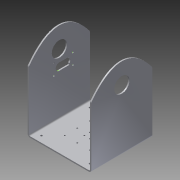
# Autodesk Inventor part: U Arms
Saved by Autodesk Inventor 2015 (Build 190159000, 159)
## iProperties
Created: 2014-05-20
Part Number: U Arms
Material: Aluminum 6061
Document SubType Name: Sheet Metal
Designer: seaha_000
Density: 2.71 g/cm^3
Sheet Metal Rule: 1/8in Aluminium
Sheet Metal Width: 6.000 in
Sheet Metal Length: 21.815 in
Sheet Metal Area: 130.893 in^2
Appearance: Aluminum - Flat
Flat Pattern Width: 15.24 cm
Flat Pattern Length: 55.4113 cm
Flat Pattern Area: 844.469 cm^2
Mass: 656.228 g
Surface Area: 1584.51 cm^2
Volume: 242.15 cm^3
Author: seaha_000
Autodesk Inventor part; units mm, degrees
ref_plane "YZ Plane" through (0, 0, 0) normal (1, 0, 0) x (0, 1, 0)
ref_plane "XZ Plane" through (0, 0, 0) normal (0, 1, 0) x (-1, 0, 0)
ref_plane "XY Plane" through (0, 0, 0) normal (0, 0, 1) x (1, 0, 0)
sketch "Sketch3" plane through (0, 0, 0) normal (0, 1, 0) x (-1, 0, 0)
  line L0 (-79.375, 76.2) -> (79.375, 76.2)
  line L1 (79.375, 76.2) -> (79.375, -76.2)
  line L2 (79.375, -76.2) -> (-79.375, -76.2)
  line L3 (-79.375, -76.2) -> (-79.375, 76.2)
  line L4 (-79.375, 76.2) -> (79.375, -76.2) construction
  line L5 (79.375, 76.2) -> (-79.375, -76.2) construction
  arc A0 (-19.05, -1.8288) -> (-19.05, 1.8288) centre (-19.05, 0) ccw
  arc A1 (-19.05, 1.8288) -> (-19.05, -1.8288) centre (-19.05, 0) ccw
  arc A2 (-6.9148, -8.7436) -> (-6.9148, -5.086) centre (-6.9148, -6.9148) ccw
  arc A3 (-6.9148, -5.086) -> (-6.9148, -8.7436) centre (-6.9148, -6.9148) ccw
  arc A4 (-6.9148, 5.086) -> (-6.9148, 8.7436) centre (-6.9148, 6.9148) ccw
  arc A5 (-6.9148, 8.7436) -> (-6.9148, 5.086) centre (-6.9148, 6.9148) ccw
  arc A6 (6.9148, 5.086) -> (6.9148, 8.7436) centre (6.9148, 6.9148) ccw
  arc A7 (6.9148, 8.7436) -> (6.9148, 5.086) centre (6.9148, 6.9148) ccw
  arc A8 (0, 17.2212) -> (0, 20.8788) centre (0, 19.05) ccw
  arc A9 (0, 20.8788) -> (0, 17.2212) centre (0, 19.05) ccw
  arc A10 (19.05, -1.8288) -> (19.05, 1.8288) centre (19.05, 0) ccw
  arc A11 (19.05, 1.8288) -> (19.05, -1.8288) centre (19.05, 0) ccw
  arc A12 (6.9148, -8.7436) -> (6.9148, -5.086) centre (6.9148, -6.9148) ccw
  arc A13 (6.9148, -5.086) -> (6.9148, -8.7436) centre (6.9148, -6.9148) ccw
  arc A14 (0, -20.8788) -> (0, -17.2212) centre (0, -19.05) ccw
  arc A15 (0, -17.2212) -> (0, -20.8788) centre (0, -19.05) ccw
  arc A16 (0, -46.236) -> (0, -42.664) centre (0, -44.45) ccw
  arc A17 (0, -42.664) -> (0, -46.236) centre (0, -44.45) ccw
  arc A18 (0, -33.536) -> (0, -29.964) centre (0, -31.75) ccw
  arc A19 (0, -29.964) -> (0, -33.536) centre (0, -31.75) ccw
  arc A20 (0, -11.565) -> (0, -7.993) centre (0, -9.779) ccw
  arc A21 (0, -7.993) -> (0, -11.565) centre (0, -9.779) ccw
  arc A22 (13.4704, -15.2564) -> (13.4704, -11.6844) centre (13.4704, -13.4704) ccw
  arc A23 (13.4704, -11.6844) -> (13.4704, -15.2564) centre (13.4704, -13.4704) ccw
  arc A24 (22.4506, -24.2366) -> (22.4506, -20.6646) centre (22.4506, -22.4506) ccw
  arc A25 (22.4506, -20.6646) -> (22.4506, -24.2366) centre (22.4506, -22.4506) ccw
  arc A26 (31.4309, -33.2169) -> (31.4309, -29.6449) centre (31.4309, -31.4309) ccw
  arc A27 (31.4309, -29.6449) -> (31.4309, -33.2169) centre (31.4309, -31.4309) ccw
  arc A28 (44.45, -1.786) -> (44.45, 1.786) centre (44.45, 0) ccw
  arc A29 (44.45, 1.786) -> (44.45, -1.786) centre (44.45, 0) ccw
  arc A30 (31.75, -1.786) -> (31.75, 1.786) centre (31.75, 0) ccw
  arc A31 (31.75, 1.786) -> (31.75, -1.786) centre (31.75, 0) ccw
  arc A32 (9.779, -1.786) -> (9.779, 1.786) centre (9.779, 0) ccw
  arc A33 (9.779, 1.786) -> (9.779, -1.786) centre (9.779, 0) ccw
  arc A34 (13.4704, 11.6844) -> (13.4704, 15.2564) centre (13.4704, 13.4704) ccw
  arc A35 (13.4704, 15.2564) -> (13.4704, 11.6844) centre (13.4704, 13.4704) ccw
  arc A36 (22.4506, 20.6646) -> (22.4506, 24.2366) centre (22.4506, 22.4506) ccw
  arc A37 (22.4506, 24.2366) -> (22.4506, 20.6646) centre (22.4506, 22.4506) ccw
  arc A38 (31.4309, 29.6449) -> (31.4309, 33.2169) centre (31.4309, 31.4309) ccw
  arc A39 (31.4309, 33.2169) -> (31.4309, 29.6449) centre (31.4309, 31.4309) ccw
  arc A40 (0, 42.664) -> (0, 46.236) centre (0, 44.45) ccw
  arc A41 (0, 46.236) -> (0, 42.664) centre (0, 44.45) ccw
  arc A42 (0, 29.964) -> (0, 33.536) centre (0, 31.75) ccw
  arc A43 (0, 33.536) -> (0, 29.964) centre (0, 31.75) ccw
  arc A44 (0, 7.993) -> (0, 11.565) centre (0, 9.779) ccw
  arc A45 (0, 11.565) -> (0, 7.993) centre (0, 9.779) ccw
  arc A46 (-13.4704, 11.6844) -> (-13.4704, 15.2564) centre (-13.4704, 13.4704) ccw
  arc A47 (-13.4704, 15.2564) -> (-13.4704, 11.6844) centre (-13.4704, 13.4704) ccw
  arc A48 (-22.4506, 20.6646) -> (-22.4506, 24.2366) centre (-22.4506, 22.4506) ccw
  arc A49 (-22.4506, 24.2366) -> (-22.4506, 20.6646) centre (-22.4506, 22.4506) ccw
  arc A50 (-31.4309, 29.6449) -> (-31.4309, 33.2169) centre (-31.4309, 31.4309) ccw
  arc A51 (-31.4309, 33.2169) -> (-31.4309, 29.6449) centre (-31.4309, 31.4309) ccw
  arc A52 (-44.45, -1.786) -> (-44.45, 1.786) centre (-44.45, 0) ccw
  arc A53 (-44.45, 1.786) -> (-44.45, -1.786) centre (-44.45, 0) ccw
  arc A54 (-31.75, -1.786) -> (-31.75, 1.786) centre (-31.75, 0) ccw
  arc A55 (-31.75, 1.786) -> (-31.75, -1.786) centre (-31.75, 0) ccw
  arc A56 (-9.779, -1.786) -> (-9.779, 1.786) centre (-9.779, 0) ccw
  arc A57 (-9.779, 1.786) -> (-9.779, -1.786) centre (-9.779, 0) ccw
  arc A58 (-13.4704, -15.2564) -> (-13.4704, -11.6844) centre (-13.4704, -13.4704) ccw
  arc A59 (-13.4704, -11.6844) -> (-13.4704, -15.2564) centre (-13.4704, -13.4704) ccw
  arc A60 (-22.4506, -24.2366) -> (-22.4506, -20.6646) centre (-22.4506, -22.4506) ccw
  arc A61 (-22.4506, -20.6646) -> (-22.4506, -24.2366) centre (-22.4506, -22.4506) ccw
  arc A62 (-31.4309, -33.2169) -> (-31.4309, -29.6449) centre (-31.4309, -31.4309) ccw
  arc A63 (-31.4309, -29.6449) -> (-31.4309, -33.2169) centre (-31.4309, -31.4309) ccw
  arc A64 (0, 50.038) -> (0, -50.038) centre (0, 0) ccw
  arc A65 (0, -50.038) -> (0, 50.038) centre (0, 0) ccw
  arc A66 (0, 6.35) -> (0, -6.35) centre (0, 0) ccw
  arc A67 (0, -6.35) -> (0, 6.35) centre (0, 0) ccw
  dimension "d185" = 158.75
  dimension "d186" = 152.4
  dimension "d187" = 1.786
  dimension "d188" = 1.786
  dimension "d189" = 1.786
  dimension "d190" = 1.786
  dimension "d191" = 1.786
  dimension "d192" = 1.786
  dimension "d193" = 1.786
  dimension "d194" = 1.8288
  dimension "d195" = 1.8288
  dimension "d196" = 1.786
  dimension "d197" = 1.786
  dimension "d198" = 1.786
  dimension "d199" = 1.8288
  dimension "d200" = 1.8288
  dimension "d201" = 1.786
  dimension "d202" = 1.786
  dimension "d203" = 1.8288
  dimension "d204" = 1.786
  dimension "d205" = 50.038
  dimension "d206" = 50.038
  dimension "d207" = 6.35
  dimension "d208" = 6.35
  dimension "d209" = 1.786
  dimension "d210" = 1.8288
  dimension "d211" = 1.786
  dimension "d212" = 1.786
  dimension "d213" = 1.8288
  dimension "d214" = 1.8288
  dimension "d215" = 1.786
  dimension "d216" = 1.786
  dimension "d217" = 1.786
  dimension "d218" = 1.8288
  dimension "d219" = 1.786
  dimension "d220" = 1.786
  dimension "d221" = 1.786
  dimension "d222" = 1.786
  dimension "d223" = 1.786
  dimension "d224" = 1.786
  dimension "d225" = 74.414
  dimension "d226" = 34.925
  dimension "d227" = 76.2
  dimension "d228" = 76.2
  dimension "d229" = 74.414
  dimension "d230" = 47.625
  dimension "d231" = 76.2
  dimension "d232" = 76.2
  dimension "d233" = 42.9831
  dimension "d234" = 47.9441
  dimension "d235" = 44.7691
  dimension "d236" = 44.7691
  dimension "d237" = 105.8449
  dimension "d238" = 47.9441
  dimension "d239" = 107.6309
  dimension "d240" = 107.6309
  dimension "d241" = 51.9634
  dimension "d242" = 56.9244
  dimension "d243" = 53.7494
  dimension "d244" = 53.7494
  dimension "d245" = 96.8646
  dimension "d246" = 56.9244
  dimension "d247" = 98.6506
  dimension "d248" = 98.6506
  measures "d185" distance of L1.end L2.end
  measures "d186" distance of L0.end L1.end
  measures "d187" radius of A29
  measures "d188" radius of A28
  measures "d189" radius of A30
  measures "d190" radius of A38
  measures "d191" radius of A26
  measures "d192" radius of A36
  measures "d193" radius of A24
  measures "d194" radius of A11
  measures "d195" radius of A10
  measures "d196" radius of A34
  measures "d197" radius of A22
  measures "d198" radius of A32
  measures "d199" radius of A6
  measures "d200" radius of A12
  measures "d201" radius of A40
  measures "d202" radius of A42
  measures "d203" radius of A8
  measures "d204" radius of A44
  measures "d205" radius of A64
  measures "d206" radius of A65
  measures "d207" radius of A67
  measures "d208" radius of A66
  measures "d209" radius of A20
  measures "d210" radius of A14
  measures "d211" radius of A18
  measures "d212" radius of A16
  measures "d213" radius of A4
  measures "d214" radius of A2
  measures "d215" radius of A56
  measures "d216" radius of A46
  measures "d217" radius of A58
  measures "d218" radius of A0
  measures "d219" radius of A48
  measures "d220" radius of A60
  measures "d221" radius of A50
  measures "d222" radius of A62
  measures "d223" radius of A54
  measures "d224" radius of A52
  measures "d225" distance from line of A28.end L0
  measures "d226" distance from line of A28.end L1
  measures "d227" distance from line of A29.centre L0
  measures "d228" distance from line of A28.centre L0
  measures "d229" distance from line of A30.end L0
  measures "d230" distance from line of A30.end L1
  measures "d231" distance from line of A31.centre L0
  measures "d232" distance from line of A30.centre L0
  measures "d233" distance from line of A38.end L0
  measures "d234" distance from line of A38.end L1
  measures "d235" distance from line of A39.centre L0
  measures "d236" distance from line of A38.centre L0
  measures "d237" distance from line of A26.end L0
  measures "d238" distance from line of A26.end L1
  measures "d239" distance from line of A27.centre L0
  measures "d240" distance from line of A26.centre L0
  measures "d241" distance from line of A36.end L0
  measures "d242" distance from line of A36.end L1
  measures "d243" distance from line of A37.centre L0
  measures "d244" distance from line of A36.centre L0
  measures "d245" distance from line of A24.end L0
  measures "d246" distance from line of A24.end L1
  measures "d247" distance from line of A25.centre L0
  measures "d248" distance from line of A24.centre L0
extrude "Plate3" add sketch "Sketch3" along normal blind 3.175 contours L0 L1 L2 L3 | A65 A64
sketch "Sketch4" plane through (76.2, 0, -76.2) normal (1, 0, 0) x (0, 1, 0)
  line L0 (0, 152.4) -> (0, 0)
  line L1 (0, 0) -> (203.2, 0)
  line L2 (203.2, 0) -> (203.2, 152.4)
  line L3 (203.2, 152.4) -> (0, 152.4)
  constraints: 6 end point, 1 horizontal, 1 perpendicular, 1 vertical
edge flange "Flange2" height 203.2 angle 90 thickness 3.175 bend radius 3.175 thickness toward (1, 0, 0) relief tear relief width 3.175 relief depth 1.5875 corner gap 3.175 corner form 0 edges at (79.375, 3.175, 0) (-79.375, 3.175, 0) wall of the first edge with corners at (76.2, 0, 76.2) (76.2, 0, -76.2) (76.2, 203.2, -76.2) (76.2, 203.2, 76.2)
bend "Bend2"
corner "Corner2"
sketch "Sketch5" plane through (79.375, 203.2, 76.2) normal (1, 0, 0) x (0, 0, -1)
  line L0 (152.4, 0) -> (152.4, -196.85) projected
  line L1 (0, 0) -> (152.4, 0) projected
  line L2 (0, -196.85) -> (0, 0) projected
  line L3 (0, -50.8) -> (152.4, -50.8)
  spline S0 degree 2 poles (0, -50.8) (76.2, 50.8) (152.4, -50.8) knots 0 0 0 1 1 1
  circle A0 centre (76.2, -50.8) radius 19.05
  point P0 (76.2, -203.2)
  point P1 (76.2, 0)
  dimension "d370" = 152.4
  dimension "d371" = 50.8
  dimension "d372" = 38.1
  constraints: 2 end point, 2 midpoint, 2 point on line, 1 centre point, 3 other
  measures "d370" distance of L3.start L3.end
  measures "d371" distance from line of L0.start L3
  measures "d372" diameter of A0
extrude "Cut1" cut sketch "Sketch5" against normal through all contours L0 S0 L1 | S0 L2 L1 | A0 L3 | L3 A0
fillet "Corner Round1" radius 6.35 4 edges at (-77.7875, 152.4, -76.2) (77.7875, 152.4, -76.2) (-77.7875, 152.4, 76.2) (77.7875, 152.4, 76.2)
sketch "Sketch6" plane through (0, 0, 0) normal (0, -1, 0) x (1, 0, 0)
  circle A0 centre (0, 0) radius 6.35 projected
  line L0 (73.025, 76.2) -> (-73.025, 76.2) projected
  arc A1 (60.4833, -62.9154) -> (60.5748, -62.9153) centre (60.5282, -60.5282) ccw
  arc A2 (60.5748, -62.9153) -> (60.4833, -62.9154) centre (60.5282, -60.5282) ccw
  arc A3 (60.4833, 58.141) -> (60.5748, 58.1411) centre (60.5282, 60.5282) ccw
  arc A4 (60.5748, 58.1411) -> (60.4833, 58.141) centre (60.5282, 60.5282) ccw
  arc A5 (-60.5731, 58.141) -> (-60.4816, 58.1411) centre (-60.5282, 60.5282) ccw
  arc A6 (-60.4816, 58.1411) -> (-60.5731, 58.141) centre (-60.5282, 60.5282) ccw
  arc A7 (-60.5731, -62.9154) -> (-60.4816, -62.9153) centre (-60.5282, -60.5282) ccw
  arc A8 (-60.4816, -62.9153) -> (-60.5731, -62.9154) centre (-60.5282, -60.5282) ccw
  line L1 (77.0001, -77.0001) -> (77.0001, 77.0001)
  line L2 (77.0001, 77.0001) -> (-77.0001, 77.0001)
  line L3 (-77.0001, 77.0001) -> (-77.0001, -77.0001)
  line L4 (-77.0001, -77.0001) -> (77.0001, -77.0001)
  arc A9 (-26.6715, -70.6634) -> (63.3445, -41.1358) centre (0, 0) ccw
  arc A10 (63.3445, -41.1358) -> (-26.6715, -70.6634) centre (0, 0) ccw
  dimension "d376" = 75.5293
  dimension "d377" = 75.5293
  dimension "d378" = 2.3876
  dimension "d379" = 2.3876
  dimension "d380" = 2.3876
  dimension "d381" = 2.3876
  dimension "d382" = 2.3876
  dimension "d383" = 2.3876
  dimension "d384" = 2.3876
  dimension "d385" = 2.3876
  dimension "d386" = 154.0002
  dimension "d387" = 154.0002
  dimension "d388" = 77.0001
  dimension "d389" = 77.0001
  dimension "d390" = 60.5282
  dimension "d391" = 60.5282
  dimension "d392" = 60.5282
  dimension "d393" = 60.5282
  dimension "d394" = 60.5282
  dimension "d395" = 60.5282
  dimension "d396" = 60.5282
  dimension "d397" = 60.5282
  dimension "d398" = 117.3358
  dimension "d399" = 18.0589
  dimension "d400" = 139.1153
  dimension "d401" = 18.0589
  dimension "d402" = 139.1153
  constraints: 20 point on circle, 10 centre point, 8 end point, 5 concentric, 2 horizontal, 2 vertical, 1 coincident
  measures "d376" radius of A9
  measures "d377" radius of A10
  measures "d378" radius of A3
  measures "d379" radius of A4
  measures "d380" radius of A1
  measures "d381" radius of A2
  measures "d382" radius of A7
  measures "d383" radius of A8
  measures "d384" radius of A5
  measures "d385" radius of A6
  measures "d386" distance of L1.end L2.end
  measures "d387" distance of L1.start L1.end
  measures "d388" distance from line of L1 A10.centre
  measures "d389" distance from line of L4 A9.centre
  measures "d390" horizontal distance of A10.centre A5.centre
  measures "d391" horizontal distance of A9.centre A3.centre
  measures "d392" horizontal distance of A9.centre A8.centre
  measures "d393" horizontal distance of A1.centre A9.centre
  measures "d394" horizontal distance of A9.centre A7.centre
  measures "d395" horizontal distance of A9.centre A1.centre
  measures "d396" horizontal distance of A3.centre A10.centre
  measures "d397" horizontal distance of A9.centre A5.centre
  measures "d398" distance from line of A9.end L0
  measures "d399" distance from line of A3.end L0
  measures "d400" distance from line of A1.end L0
  measures "d401" distance from line of A5.end L0
  measures "d402" distance from line of A7.end L0
hole "Hole1" at (-60.5282, 0, 60.5282) at (60.5282, 0, 60.5282) at (60.5282, 0, -60.5282) at (-60.5282, 0, -60.5282) direction (0, 1, 0) diameter 4.826 end through all
sketch "Sketch7" plane through (-79.375, 6.35, -76.2) normal (-1, 0, 0) x (0, 0, 1)
  circle A0 centre (76.2, 146.05) radius 19.05 construction
  line L0 (0, 0) -> (152.4, 0) construction
  line L1 (152.4, 143.9189) -> (152.4, 0) construction
  line L2 (0, 0) -> (0, 143.9189) construction
  line L3 (76.2, 196.85) -> (76.2, 0) construction
  line L4 (152.4, 0) -> (0, 0) construction
  line L5 (76.2, 146.05) -> (152.0317, 146.05) construction
  line L6 (76.2, 146.05) -> (0.3683, 146.05) construction
  circle A1 centre (76.2, 107.95) radius 9.2964
  line L7 (76.2, 107.95) -> (152.4, 107.95) construction
  line L8 (76.2, 107.95) -> (0, 107.95) construction
  circle A2 centre (55.2, 107.95) radius 6.2103
  line L9 (73.4328, 99.075) -> (51.346, 99.075)
  line L10 (51.346, 99.075) -> (51.346, 116.825)
  line L11 (51.346, 116.825) -> (73.4328, 116.825)
  line L12 (73.4328, 116.825) -> (73.4328, 99.075)
  point P0 (76.2, -6.35)
  dimension "d410" = 18.5928
  dimension "d411" = 38.1
  dimension "d412" = 12.4206
  dimension "d413" = 21
  dimension "d414" = 8.875
  dimension "d415" = 8.875
  dimension "d416" = 3.854
  constraints: 18 end point, 6 point on line, 2 horizontal, 2 parallel, 2 perpendicular, 1 centre point, 1 midpoint, 9 other
  measures "d411" distance from line of L5 L7.start
  measures "d412" diameter of A2
  measures "d413" distance of L7.start A2.centre
  measures "d414" distance from line of A2.centre L9
  measures "d415" distance from line of A2.centre L11
  measures "d416" distance from line of A2.centre L10
extrude "Cut2" cut sketch "Sketch7" against normal blind 3.175
sketch "Sketch8" plane through (-79.375, 6.35, -76.2) normal (-1, 0, 0) x (0, 0, 1)
  circle A0 centre (42.3239, 121.4153) radius 1.8288
  circle A1 centre (42.3239, 94.4745) radius 1.8288
  circle A2 centre (90.084, 94.4745) radius 1.8288
  circle A3 centre (90.084, 121.4153) radius 1.8288
  line L0 (85.2015, 117.95) -> (47.2015, 117.95)
  line L1 (85.8629, 98.2) -> (46.54, 98.2)
  line L2 (46.2015, 116.95) -> (46.2015, 98.95)
  line L3 (85.9515, 117.6114) -> (85.9515, 98.2886)
  point P0 (76.2, -6.35)
  constraints: 8 end point, 4 centre point
hole "Hole2" at (-79.375, 127.7653, -33.8761) at (-79.375, 100.8245, -33.8761) at (-79.375, 100.8245, 13.884) direction (1, 0, 0) diameter 3.6576 depth 3.175 tip angle 118 clearance for "Flat Head Machine Screw (82)" size "#6" standard "Ansi Unified Screw Threads"
hole "Hole3" at (-79.375, 127.7653, 13.884) direction (1, 0, 0) diameter 2.6416 depth 10.9728 tip angle 118 thread size "6-32 UNC" class "2B" standard "ANSI Unified Screw Threads"
sketch "Sketch9" plane through (0, 3.175, 0) normal (0, 1, 0) x (1, 0, 0)
  circle A0 centre (60.5282, 60.5282) radius 2.413 projected
  circle A1 centre (-60.5282, -60.5282) radius 2.413 projected
  circle A2 centre (60.5282, -60.5282) radius 2.413 projected
  circle A3 centre (-60.5282, 60.5282) radius 2.413 projected
  line L0 (-73.025, 76.2) -> (-73.025, -76.2) projected
  line L1 (73.025, -76.2) -> (-73.025, -76.2) projected
  line L2 (73.025, -76.2) -> (73.025, 76.2) projected
  line L3 (-73.025, 76.2) -> (73.025, 76.2) projected
  circle A4 centre (0, 0) radius 6.35 projected
  circle A5 centre (0, 19.05) radius 1.8288 projected
  circle A6 centre (-6.9148, 6.9148) radius 1.8288 projected
  circle A7 centre (-19.05, 0) radius 1.8288 projected
  circle A8 centre (0, -19.05) radius 1.8288 projected
  circle A9 centre (-6.9148, -6.9148) radius 1.8288 projected
  circle A10 centre (6.9148, -6.9148) radius 1.8288 projected
  circle A11 centre (6.9148, 6.9148) radius 1.8288 projected
  circle A12 centre (19.05, 0) radius 1.8288 projected
  circle A13 centre (31.4309, 31.4309) radius 1.786 projected
  circle A14 centre (22.4506, 22.4506) radius 1.786 projected
  circle A15 centre (13.4704, 13.4704) radius 1.786 projected
  circle A16 centre (9.779, 0) radius 1.786 projected
  circle A17 centre (31.75, 0) radius 1.786 projected
  circle A18 centre (44.45, 0) radius 1.786 projected
  circle A19 centre (31.4309, -31.4309) radius 1.786 projected
  circle A20 centre (22.4506, -22.4506) radius 1.786 projected
  circle A21 centre (13.4704, -13.4704) radius 1.786 projected
  circle A22 centre (0, -9.779) radius 1.786 projected
  circle A23 centre (0, -31.75) radius 1.786 projected
  circle A24 centre (0, -44.45) radius 1.786 projected
  circle A25 centre (-31.4309, -31.4309) radius 1.786 projected
  circle A26 centre (-22.4506, -22.4506) radius 1.786 projected
  circle A27 centre (-13.4704, -13.4704) radius 1.786 projected
  circle A28 centre (-9.779, 0) radius 1.786 projected
  circle A29 centre (-31.75, 0) radius 1.786 projected
  circle A30 centre (-44.45, 0) radius 1.786 projected
  circle A31 centre (-31.4309, 31.4309) radius 1.786 projected
  circle A32 centre (-22.4506, 22.4506) radius 1.786 projected
  circle A33 centre (-13.4704, 13.4704) radius 1.786 projected
  circle A34 centre (0, 9.779) radius 1.786 projected
  circle A35 centre (0, 31.75) radius 1.786 projected
  circle A36 centre (0, 44.45) radius 1.786 projected
extrude "Extrusion1" add sketch "Sketch9" against normal up to surface (3.175 mm away) contours A4 | A5 | A7 | A8 | A12 | A14 | A15 | A16 | A18 | A20 | A21 | A22 | A24 | A26 | A27 | A28 | A30 | A32 | A33 | A34 | A36
equation "\"d373\" = Thickness"
equation "\"d408\" = Thickness"
equation "\"d415\" = d414"
equation "\"d417\" = Thickness"
equation "\"d424\" = Thickness"
equation "\"d360\" = BendReliefWidth"
equation "\"d361\" = BendReliefDepth"
equation "\"d362\" = MinimumRemnant"
equation "\"d363\" = BendRadius"
equation "\"d366\" = BendRadius"
equation "\"d367\" = CornerReliefSize"
equation "\"d368\" = GapSize"
equation "\"d369\" = JacobiRadiusSize"
equation "\"BendRadius\" = Thickness"
equation "\"BendReliefWidth\" = Thickness"
equation "\"BendReliefDepth\" = 0.5 * Thickness"
equation "\"CornerReliefSize\" = 4 * Thickness"
equation "\"MinimumRemnant\" = 2 * Thickness"
equation "\"TransitionRadius\" = BendRadius"
equation "\"JacobiRadiusSize\" = BendRadius"
equation "\"GapSize\" = Thickness"
equation "\"d174\" = BendRadius"
equation "\"d359\" = BendRadius"
equation "\"Thickness\" = 3.175"
body "Solid2"
